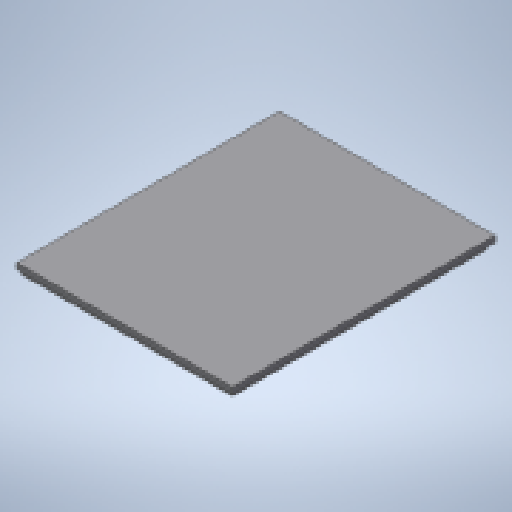
# Autodesk Inventor part: TAPITA LA REAL AHORA SI
Saved by Autodesk Inventor 2023 (Build 270158000, 158)
## iProperties
Created: 2022-10-19
Part Number: TAPITA LA REAL AHORA SI
Material: Generic
Document SubType Name: Modeling
Designer: Kimberly
Density: 1 g/cm^3
Appearance: Default
Author: Kimberly
Autodesk Inventor part; units mm, degrees
ref_plane "YZ Plane" through (0, 0, 0) normal (1, 0, 0) x (0, 1, 0)
ref_plane "XZ Plane" through (0, 0, 0) normal (0, 1, 0) x (-1, 0, 0)
ref_plane "XY Plane" through (0, 0, 0) normal (0, 0, 1) x (1, 0, 0)
sketch "Sketch5" plane through (0, 0, 0) normal (0, 1, 0) x (-1, 0, 0)
  line L0 (0, 0) -> (108, 0)
  line L1 (108, 0) -> (108, -130)
  line L2 (108, -130) -> (0, -130)
  line L3 (0, -130) -> (0, 0)
  dimension "d16" = 108
  dimension "d17" = 130
  constraints: 8 end point, 2 parallel, 1 horizontal, 1 perpendicular
  measures "d16" distance of L1.end L2.end
  measures "d17" distance of L0.end L1.end
extrude "Extrusion4" add sketch "Sketch5" along normal blind 6
sketch "Sketch7" plane through (-108, 0, 0) normal (0, 0, 1) x (1, 0, 0)
  line L0 (0, 0) -> (108, 0) projected
  line L1 (108, 0) -> (108, 6) projected
  line L2 (0, 6) -> (108, 6) projected
  line L3 (0, 0) -> (0, 6) projected
  line L4 (108, 6) -> (0, 6)
  line L5 (0, 6) -> (0, 3)
  line L6 (108, 4) -> (108, 6)
  line L7 (108, 3) -> (0, 3)
  dimension "d35" = 3
  constraints: 8 end point, 2 perpendicular, 2 point on line, 1 horizontal, 1 midpoint, 1 parallel
  measures "d35" distance between parallel lines of L7 L2
extrude "Extrusion6" add sketch "Sketch7" along normal blind 2 and the other way blind 132 contours L3 L2 L1 L7
sketch "Sketch8" plane through (0, 0, 0) normal (1, 0, 0) x (0, 0, -1)
  line L0 (0, 0) -> (0, 3) projected
  line L1 (0, 0) -> (130, 0) projected
  line L2 (130, 0) -> (130, 3) projected
  line L3 (130, 3) -> (132, 3) projected
  line L4 (132, 6) -> (-2, 6) projected
  line L5 (-2, 3) -> (-2, 6) projected
  line L6 (0, 3) -> (130, 3)
  line L7 (132, 6) -> (132, 3) projected
  line L8 (-2, 3) -> (0, 3) projected
  constraints: 2 end point, 1 collinear, 1 point on line
extrude "Extrusion7" add sketch "Sketch8" along normal blind 2 contours L8 L5 L4 L7 L3 L6
body "Solid2"
